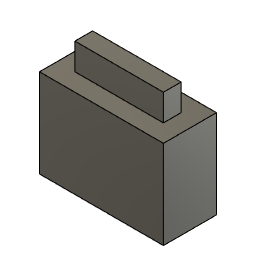
Spacer v1 (Autodesk Fusion 360 design; units mm, degrees)
Autodesk Fusion 360 part; units mm, degrees
sketch "Sketch1" plane through (0, 0, 0) normal (0, 1, 0) x (1, 0, 0)
  line L0 (0, 0) -> (14, 0)
  line L1 (14, 0) -> (14, 6)
  line L2 (14, 6) -> (0, 6)
  line L3 (0, 6) -> (0, 0)
  dimension "d1" = 14
  dimension "d2" = 6
  constraint horizontal L0
  constraint vertical L1
  constraint horizontal L2
  constraint vertical L3
  constraint coincident L0.start L3.end
  measures "d1" distance of L0.start L0.end
  measures "d2" distance of L0.start L2.end
extrude "Extrude1" add sketch "Sketch1" along normal blind 10
sketch "Sketch2" plane through (0, 10, 0) normal (0, 1, 0) x (-1, 0, 0)
  line L0 (0, -6) -> (0, 0)
  line L1 (0, 0) -> (-14, 0)
  line L2 (-14, 0) -> (-14, -6)
  line L3 (-14, -6) -> (0, -6)
  line L4 (-2, -4) -> (-12, -4)
  line L5 (-12, -4) -> (-12, -2)
  line L6 (-12, -2) -> (-2, -2)
  line L7 (-2, -2) -> (-2, -4)
  dimension "d5" = 2
  dimension "d6" = 2
  dimension "d7" = 2
  dimension "d8" = 2
  constraint horizontal L4
  constraint vertical L5
  constraint horizontal L6
  constraint vertical L7
  measures "d5" distance of L0 L7
  measures "d6" distance of L2 L5
  measures "d7" distance of L3 L4
  measures "d8" distance of L1 L6
extrude "Extrude2" add sketch "Sketch2" along normal blind 3 contours L4 L5 L6 L7
